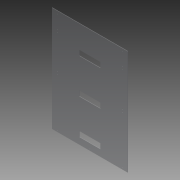
# Autodesk Inventor part: GE-13010
Saved by Autodesk Inventor 2013 (Build 170138000, 138)
## iProperties
Created: 2012-12-31
Part Number: GE-13010
Material: Polycarbonate, Clear
Document SubType Name: Modeling
Designer: Phillip
Density: 1 g/cm^3
Author: Phillip
Autodesk Inventor part; units mm, degrees
ref_plane "YZ Plane" through (0, 0, 0) normal (1, 0, 0) x (0, 1, 0)
ref_plane "XZ Plane" through (0, 0, 0) normal (0, 1, 0) x (-1, 0, 0)
ref_plane "XY Plane" through (0, 0, 0) normal (0, 0, 1) x (1, 0, 0)
sketch "Sketch1" plane through (0, 0, 0) normal (0, 0, 1) x (1, 0, 0)
  line L0 (-546.1, -758.825) -> (546.1, -758.825)
  line L1 (546.1, -758.825) -> (546.1, 758.825)
  line L2 (546.1, 758.825) -> (-546.1, 758.825)
  line L3 (-546.1, 758.825) -> (-546.1, -758.825)
  line L4 (-546.1, -758.825) -> (546.1, 758.825) construction
  line L5 (546.1, -758.825) -> (-546.1, 758.825) construction
  point P0 (0, 0)
  dimension "d0" = 1092.2
  dimension "d1" = 1517.65
  constraints: 12 end point, 2 midpoint, 2 parallel, 1 horizontal, 1 perpendicular
  measures "d0" distance of L2.end L1.end
  measures "d1" distance of L1.end L0.end
extrude "Extrusion1" add sketch "Sketch1" against normal blind 6.35
sketch "Sketch2" plane through (0, 0, 0) normal (0, 0, 1) x (1, 0, 0)
  line L0 (546.1, 758.825) -> (-546.1, 758.825) projected
  line L1 (-546.1, 758.825) -> (-546.1, -758.825) projected
  line L2 (-152.4, 352.425) -> (152.4, 352.425)
  line L3 (152.4, 352.425) -> (152.4, 428.625)
  line L4 (152.4, 428.625) -> (-152.4, 428.625)
  line L5 (-152.4, 428.625) -> (-152.4, 352.425)
  line L6 (-152.4, -155.575) -> (152.4, -155.575)
  line L7 (152.4, -155.575) -> (152.4, -79.375)
  line L8 (152.4, -79.375) -> (-152.4, -79.375)
  line L9 (-152.4, -79.375) -> (-152.4, -155.575)
  line L10 (-152.4, -663.575) -> (152.4, -663.575)
  line L11 (152.4, -663.575) -> (152.4, -587.375)
  line L12 (152.4, -587.375) -> (-152.4, -587.375)
  line L13 (-152.4, -587.375) -> (-152.4, -663.575)
  point P0 (0, 0)
  dimension "d4" = 330.2
  dimension "d5" = 406.4
  dimension "d6" = 838.2
  dimension "d7" = 914.4
  dimension "d8" = 1346.2
  dimension "d9" = 1422.4
  dimension "d10" = 393.7
  dimension "d11" = 698.5
  constraints: 24 end point, 6 parallel, 4 collinear, 3 horizontal, 3 perpendicular
  measures "d4" distance between parallel lines of L4 L0
  measures "d5" distance between parallel lines of L2 L0
  measures "d6" distance between parallel lines of L8 L0
  measures "d7" distance between parallel lines of L6 L0
  measures "d8" distance between parallel lines of L12 L0
  measures "d9" distance between parallel lines of L10 L0
  measures "d10" distance between parallel lines of L5 L1
  measures "d11" distance between parallel lines of L3 L1
extrude "Extrusion2" cut sketch "Sketch2" against normal up to next
sketch "Sketch3" plane through (0, 0, 0) normal (0, 0, 1) x (1, 0, 0)
  line L0 (546.1, 758.825) -> (-546.1, 758.825) projected
  line L1 (-546.1, 758.825) -> (-546.1, -758.825) projected
  point P0 (0, 0)
  point P1 (-469.9, 720.725)
  point P2 (-469.9, 530.225)
  point P3 (-469.9, 492.379)
  point P4 (-469.9, -3.175)
  point P5 (-469.9, -41.021)
  point P6 (-469.9, -733.425)
  point P7 (469.9, 720.725)
  point P8 (469.9, 530.225)
  point P9 (469.9, 492.379)
  point P10 (469.9, -3.175)
  point P11 (469.9, -41.021)
  point P12 (469.9, -733.425)
  point P13 (0, -733.425)
  dimension "d14" = 38.1
  dimension "d16" = 1016
  dimension "d17" = 228.6
  dimension "d18" = 266.446
  dimension "d20" = 762
  dimension "d21" = 799.846
  dimension "d22" = 1492.25
  dimension "d23" = 76.2
  dimension "d24" = 1016
  dimension "d32" = 546.1
  constraints: 8 vertical alignment, 7 horizontal alignment
  measures "d14" distance from line of point (-469.9, 720.725) L0
  measures "d16" distance from line of point (469.9, 720.725) L1
  measures "d17" distance from line of point (-469.9, 530.225) L0
  measures "d18" distance from line of point (-469.9, 492.379) L0
  measures "d20" distance from line of point (-469.9, -3.175) L0
  measures "d21" distance from line of point (-469.9, -41.021) L0
  measures "d22" distance from line of point (-469.9, -733.425) L0
  measures "d23" distance from line of point (-469.9, -733.425) L1
  measures "d24" distance from line of point (469.9, -733.425) L1
  measures "d32" distance from line of point (0, -733.425) L1
hole "Hole1" at (-469.9, 720.725, 0) at (-469.9, 530.225, 0) at (-469.9, 492.379, 0) at (-469.9, -3.175, 0) at (-469.9, -41.021, 0) at (-469.9, -733.425, 0) at (469.9, 720.725, 0) at (469.9, 530.225, 0) at (469.9, 492.379, 0) at (469.9, -3.175, 0) at (469.9, -41.021, 0) at (469.9, -733.425, 0) at (0, -733.425, 0) direction (0, 0, -1) diameter 9.652 end through all
body "Solid1"
